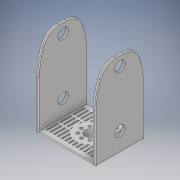
# Autodesk Inventor part: Wheel Case V3
Saved by Autodesk Inventor 2019 (Build 230136000, 136)
## iProperties
Created: 2018-12-01
Part Number: Wheel Case V3
Material: Generic
Document SubType Name: Modeling
Designer: Ashley
Density: 1 g/cm^3
Appearance: Default
Author: Ashley
Autodesk Inventor part; units mm, degrees
ref_plane "YZ Plane" through (0, 0, 0) normal (1, 0, 0) x (0, 1, 0)
ref_plane "XZ Plane" through (0, 0, 0) normal (0, 1, 0) x (-1, 0, 0)
ref_plane "XY Plane" through (0, 0, 0) normal (0, 0, 1) x (1, 0, 0)
sketch "Sketch1" plane through (0, 0, 0) normal (0, 1, 0) x (-1, 0, 0)
  line L0 (40, 32.5) -> (-40, 32.5)
  line L1 (-40, 32.5) -> (-40, -32.5)
  line L2 (-40, -32.5) -> (40, -32.5)
  line L3 (40, -32.5) -> (40, 32.5)
  line L4 (40, 32.5) -> (-40, -32.5) construction
  line L5 (-40, 32.5) -> (40, -32.5) construction
  point P0 (0, 0)
  dimension "d0" = 80
  dimension "d1" = 65
  constraints: 12 end point, 2 midpoint, 2 parallel, 1 horizontal, 1 perpendicular
  measures "d0" distance of L1.end L2.end
  measures "d1" distance of L0.end L1.end
extrude "Top Base Extrusion" add sketch "Sketch1" along normal blind 4
sketch "Sketch2" plane through (0, 4, 0) normal (0, 1, 0) x (1, 0, 0)
  line L0 (-40, -32.5) -> (40, -32.5) construction
  line L1 (40, -32.5) -> (40, 32.5) construction
  line L2 (-40, 32.5) -> (-40, -32.5) construction
  line L3 (-40, 32.5) -> (-36, 32.5)
  line L4 (-36, 32.5) -> (-36, -32.5)
  line L5 (-36, -32.5) -> (-40, -32.5)
  line L6 (-40, -32.5) -> (-40, 32.5)
  line L7 (40, 32.5) -> (36, 32.5)
  line L8 (36, 32.5) -> (36, -32.5)
  line L9 (36, -32.5) -> (40, -32.5)
  line L10 (40, -32.5) -> (40, 32.5)
  point P0 (0, 0)
  dimension "d4" = 4
  dimension "d5" = 4
  constraints: 16 end point, 4 parallel, 2 horizontal, 2 perpendicular, 2 point on line
  measures "d4" distance between parallel lines of L4 L2
  measures "d5" distance between parallel lines of L1 L8
extrude "Side Extrusions" add sketch "Sketch2" along normal blind 110
sketch "Sketch3" plane through (40, 0, 32.5) normal (1, 0, 0) x (0, 0, -1)
  circle A0 centre (32.5, 101.5) radius 7.1
  circle A1 centre (32.5, 26.5) radius 7
  line L0 (65, 0) -> (65, 114) construction
  line L1 (0, 114) -> (65, 114) construction
  line L2 (0, 0) -> (0, 114) construction
  line L3 (0, 4) -> (65, 4) construction
  point P0 (32.5, 0)
  dimension "d8" = 14.2
  dimension "d11" = 101.5
  dimension "d43" = 75
  dimension "d44" = 14
  dimension "d45" = 65
  dimension "d46" = 32.5
  dimension "d47" = 32.5
  dimension "d48" = 32.5
  dimension "d49" = 12.5
  dimension "d50" = 22.5
  constraints: 2 centre point
  measures "d8" diameter of A0
  measures "d11" distance of point (32.5, 0) A0.centre
  measures "d43" distance of A1.centre A0.centre
  measures "d44" diameter of A1
  measures "d45" distance between parallel lines of L2 L0
  measures "d46" distance from line of L0 A0.centre
  measures "d47" distance from line of L2 A0.centre
  measures "d48" distance from line of L0 A1.centre
  measures "d49" distance from line of A0.centre L1
  measures "d50" distance from line of A1.centre L3
extrude "Wheel Axel Hole" cut sketch "Sketch3" against normal up to surface (80 mm away)
sketch "Sketch4" plane through (0, 0, 0) normal (0, -1, 0) x (1, 0, 0)
  circle A0 centre (0, 0) radius 7.1
  circle A1 centre (0, 0) radius 16
  dimension "d16" = 14.2
  dimension "d17" = 32
  constraints: 2 centre point, 2 coincident
  measures "d16" diameter of A0
  measures "d17" diameter of A1
extrude "Chain Interferance Extrusion" add sketch "Sketch4" along normal blind 6
sketch "Sketch5" plane through (0, 0, 0) normal (0, -1, 0) x (1, 0, 0)
  circle A0 centre (0, 0) radius 7.1 construction
  circle A1 centre (0, 0) radius 7.1
  constraints: 1 centre point, 1 coincident, 1 concentric
extrude "Top Center Bearing Hole" cut sketch "Sketch5" against normal up to surface (4 mm away)
sketch "Sketch7" plane through (0, -6, 0) normal (0, -1, 0) x (1, 0, 0)
  circle A0 centre (0, 0) radius 7.1 construction
  circle A1 centre (0, 11.314) radius 2.05
  circle A2 centre (-8.0002, 8.0002) radius 2.05
  circle A3 centre (-11.314, 0) radius 2.05
  circle A4 centre (-8.0002, -8.0002) radius 2.05
  circle A5 centre (0, -11.314) radius 2.05
  circle A6 centre (8.0002, -8.0002) radius 2.05
  circle A7 centre (11.314, 0) radius 2.05
  circle A8 centre (8.0002, 8.0002) radius 2.05
  dimension "d23" = 4.1
  dimension "d24" = 11.314
  dimension "d27" = 360
  constraints: 8 centre point, 17 other
  measures "d23" diameter of A1
  measures "d24" distance of A0.centre A1.centre
extrude "Sprocket Screws Holes" cut sketch "Sketch7" against normal up to next
sketch "Sketch8" plane through (40, 0, 32.5) normal (1, 0, 0) x (0, 0, -1)
  line L0 (65, 0) -> (65, 114) construction
  line L1 (0, 114) -> (65, 114) construction
  line L2 (0, 0) -> (0, 114) construction
  line L3 (65, 91.5) -> (52.0096, 114)
  line L4 (65, 114) -> (0, 114) construction
  line L5 (65, 91.5) -> (90.9808, 91.5) construction
  line L6 (0, 91.5) -> (34.6363, 91.5) construction
  line L7 (0, 91.5) -> (44.4453, 91.5) construction
  line L8 (0, 91.5) -> (12.9904, 114)
  line L9 (65, 91.5) -> (65, 114)
  line L10 (52.0096, 114) -> (65, 114)
  line L11 (12.9904, 114) -> (0, 114)
  line L12 (0, 91.5) -> (0, 114)
  line L13 (0, 91.5) -> (-31.251, 91.5) construction
  point P0 (32.5, 0)
  dimension "d32" = 120
  dimension "d51" = 120
  constraints: 20 end point, 5 point on line, 3 collinear, 3 horizontal, 1 equal length, 1 perpendicular
  measures "d32" angle of L5 L3
  measures "d51" angle of L13 L8
extrude "Side Corners Cut" cut sketch "Sketch8" against normal up to surface (80 mm away)
fillet "Fillet1" radius 95 4 edges at (38, 91.5, 32.5) (-38, 91.5, 32.5) (38, 91.5, -32.5) (-38, 91.5, -32.5)
fillet "Fillet2" radius 23 4 edges at (38, 114, 19.5096) (38, 114, -19.5096) (-38, 114, -19.5096) (-38, 114, 19.5096)
fillet "Fillet3" radius 3 4 edges at (0, 0, -32.5) (-40, 0, 0) (40, 0, 0) (0, 0, 32.5)
fillet "Fillet4" radius 3 1 edges at (-16, 0, 0)
fillet "Fillet5" radius 1 1 edges at (-16, -6, 0)
fillet "Fillet7" radius 1 34 edges at (40, 109.8726, 18.1832) (40, 114, 0) (40, 109.8726, -18.1832) (40, 82.7695, -31.0162) (40, 34.5224, -32.5) (39.1213, 0.8787, -31.6213) (40, 34.5224, 32.5) (39.1213, 0.8787, 31.6213) (40, 82.7695, 31.0162) (36, 35.0224, 32.5) (36, 109.8726, 18.1832) (36, 114, 0) (36, 109.8726, -18.1832) (36, 82.7695, -31.0162) (36, 35.0224, -32.5) (36, 82.7695, 31.0162) (-36, 109.8726, 18.1832) (-36, 114, 0) (-36, 109.8726, -18.1832) (-36, 82.7695, -31.0162) (-36, 35.0224, -32.5) (-36, 35.0224, 32.5) (-36, 82.7695, 31.0162) (-40, 34.5224, 32.5) (-39.1213, 0.8787, 31.6213) (-40, 109.8726, 18.1832) (-40, 114, 0) (-40, 109.8726, -18.1832) (-40, 82.7695, -31.0162) (-40, 34.5224, -32.5) (-39.1213, 0.8787, -31.6213) (-40, 82.7695, 31.0162) (0, 4, 32.5) (0, 4, -32.5)
sketch "Sketch10" plane through (0, 0, 0) normal (0, -1, 0) x (1, 0, 0)
  line L0 (-37, 29.5) -> (37, 29.5) construction
  line L1 (-37, -29.5) -> (-37, 29.5) construction
  line L2 (37, -29.5) -> (-37, -29.5) construction
  line L3 (37, 29.5) -> (37, -29.5) construction
  circle A0 centre (0, 0) radius 19 construction
  line L4 (33.5, -25.5) -> (31.5, -25.5)
  line L5 (31.5, -25.5) -> (31.5, -10.5)
  line L6 (31.5, -10.5) -> (33.5, -10.5)
  line L7 (33.5, -10.5) -> (33.5, -25.5)
  line L8 (31.5, -7.5) -> (31.5, 7.5)
  line L9 (33.5, 7.5) -> (33.5, -7.5)
  line L10 (31.5, 7.5) -> (33.5, 7.5)
  line L11 (33.5, -7.5) -> (31.5, -7.5)
  line L12 (31.5, 10.5) -> (31.5, 25.5)
  line L13 (33.5, 25.5) -> (33.5, 10.5)
  line L14 (31.5, 25.5) -> (33.5, 25.5)
  line L15 (33.5, 10.5) -> (31.5, 10.5)
  line L16 (26.5, -25.5) -> (26.5, -10.5)
  line L17 (28.5, -10.5) -> (28.5, -25.5)
  line L18 (26.5, -10.5) -> (28.5, -10.5)
  line L19 (28.5, -25.5) -> (26.5, -25.5)
  line L20 (26.5, -7.5) -> (26.5, 7.5)
  line L21 (28.5, 7.5) -> (28.5, -7.5)
  line L22 (26.5, 7.5) -> (28.5, 7.5)
  line L23 (28.5, -7.5) -> (26.5, -7.5)
  line L24 (26.5, 10.5) -> (26.5, 25.5)
  line L25 (28.5, 25.5) -> (28.5, 10.5)
  line L26 (26.5, 25.5) -> (28.5, 25.5)
  line L27 (28.5, 10.5) -> (26.5, 10.5)
  line L28 (21.5, -25.5) -> (21.5, -10.5)
  line L29 (23.5, -10.5) -> (23.5, -25.5)
  line L30 (21.5, -10.5) -> (23.5, -10.5)
  line L31 (23.5, -25.5) -> (21.5, -25.5)
  line L32 (21.5, -7.5) -> (21.5, 7.5)
  line L33 (23.5, 7.5) -> (23.5, -7.5)
  line L34 (21.5, 7.5) -> (23.5, 7.5)
  line L35 (23.5, -7.5) -> (21.5, -7.5)
  line L36 (21.5, 10.5) -> (21.5, 25.5)
  line L37 (23.5, 25.5) -> (23.5, 10.5)
  line L38 (21.5, 25.5) -> (23.5, 25.5)
  line L39 (23.5, 10.5) -> (21.5, 10.5)
  line L40 (16.5, -25.5) -> (16.5, -10.5)
  line L41 (18.5, -10.5) -> (18.5, -25.5)
  line L42 (16.5, -10.5) -> (18.5, -10.5)
  line L43 (18.5, -25.5) -> (16.5, -25.5)
  line L44 (16.5, 10.5) -> (16.5, 25.5)
  line L45 (16.5, 25.5) -> (18.5, 25.5)
  line L46 (18.5, 10.5) -> (16.5, 10.5)
  line L47 (18.5, 25.5) -> (18.5, 10.5)
  line L48 (13.5, 25.5) -> (11.5, 25.5)
  line L49 (11.5, 25.5) -> (11.5, 15.1245)
  line L50 (13.5, 13.3697) -> (13.5, 25.5)
  line L51 (8.5, 25.5) -> (6.5, 25.5)
  line L52 (6.5, 25.5) -> (6.5, 17.8536)
  line L53 (8.5, 16.9926) -> (8.5, 25.5)
  line L54 (3.5, 25.5) -> (1.5, 25.5)
  line L55 (1.5, 25.5) -> (1.5, 18.9407)
  line L56 (3.5, 18.6748) -> (3.5, 25.5)
  line L57 (-1.5, 25.5) -> (-3.5, 25.5)
  line L58 (-3.5, 25.5) -> (-3.5, 18.6748)
  line L59 (-1.5, 18.9407) -> (-1.5, 25.5)
  line L60 (-6.5, 25.5) -> (-8.5, 25.5)
  line L61 (-8.5, 25.5) -> (-8.5, 16.9926)
  line L62 (-6.5, 17.8536) -> (-6.5, 25.5)
  line L63 (-11.5, 25.5) -> (-13.5, 25.5)
  line L64 (-13.5, 25.5) -> (-13.5, 13.3697)
  line L65 (-11.5, 15.1245) -> (-11.5, 25.5)
  line L66 (-16.5, 25.5) -> (-18.5, 25.5)
  line L67 (-18.5, 25.5) -> (-18.5, 10.5)
  line L68 (-13, 10.5) -> (-11, 10.5)
  line L69 (-16.5, 10.5) -> (-16.5, 25.5)
  line L70 (41.0278, 0) -> (-51.455, 0) construction
  line L71 (-16.5, 10.5) -> (-18.5, 10.5)
  line L72 (-21.5, 25.5) -> (-23.5, 25.5)
  line L73 (-21.5, 10.5) -> (-21.5, 25.5)
  line L74 (-23.5, 25.5) -> (-23.5, 10.5)
  line L75 (-21.5, 10.5) -> (-23.5, 10.5)
  line L76 (-26.5, 25.5) -> (-28.5, 25.5)
  line L77 (-26.5, 10.5) -> (-26.5, 25.5)
  line L78 (-28.5, 25.5) -> (-28.5, 10.5)
  line L79 (-26.5, 10.5) -> (-28.5, 10.5)
  line L80 (-31.5, 25.5) -> (-33.5, 25.5)
  line L81 (-31.5, 10.5) -> (-31.5, 25.5)
  line L82 (-33.5, 25.5) -> (-33.5, 10.5)
  line L83 (-31.5, 10.5) -> (-33.5, 10.5)
  line L84 (-16.5, 0) -> (-16.5, -0.9905)
  line L85 (-18.5, 4.3301) -> (-18.5, 7.5)
  line L86 (-21.5, -7.5) -> (-21.5, 7.5)
  line L87 (-21.5, -7.5) -> (-23.5, -7.5)
  line L88 (-23.5, 7.5) -> (-23.5, -7.5)
  line L89 (-21.5, 7.5) -> (-23.5, 7.5)
  line L90 (-18.5, 7.5) -> (-17.4571, 7.5)
  line L91 (36.0278, 0) -> (-56.455, 0) construction
  line L92 (-28.5, 7.5) -> (-28.5, -7.5)
  line L93 (-26.5, -7.5) -> (-26.5, 7.5)
  line L94 (-26.5, 7.5) -> (-28.5, 7.5)
  line L95 (-26.5, -7.5) -> (-28.5, -7.5)
  line L96 (31.0278, 0) -> (-61.455, 0) construction
  line L97 (-33.5, 7.5) -> (-33.5, -7.5)
  line L98 (-31.5, -7.5) -> (-31.5, 7.5)
  line L99 (-31.5, 7.5) -> (-33.5, 7.5)
  line L100 (-31.5, -7.5) -> (-33.5, -7.5)
  line L101 (41.0278, -18) -> (-51.455, -18) construction
  line L102 (-23.5, -10.5) -> (-23.5, -25.5)
  line L103 (-21.5, -25.5) -> (-21.5, -10.5)
  line L104 (-21.5, -10.5) -> (-23.5, -10.5)
  line L105 (-21.5, -25.5) -> (-23.5, -25.5)
  line L106 (36.0278, -18) -> (-56.455, -18) construction
  line L107 (-28.5, -10.5) -> (-28.5, -25.5)
  line L108 (-26.5, -25.5) -> (-26.5, -10.5)
  line L109 (-26.5, -10.5) -> (-28.5, -10.5)
  line L110 (-26.5, -25.5) -> (-28.5, -25.5)
  line L111 (31.0278, -18) -> (-61.455, -18) construction
  line L112 (-33.5, -10.5) -> (-33.5, -25.5)
  line L113 (-31.5, -25.5) -> (-31.5, -10.5)
  line L114 (-31.5, -10.5) -> (-33.5, -10.5)
  line L115 (-31.5, -25.5) -> (-33.5, -25.5)
  line L116 (-16.5, -25.5) -> (-18.5, -25.5)
  line L117 (-16.5, -25.5) -> (-16.5, -10.5)
  line L118 (-18.5, -10.5) -> (-18.5, -25.5)
  line L119 (-16.5, -10.5) -> (-18.5, -10.5)
  arc A1 (-17.4571, 7.5) -> (-18.5, 4.3301) centre (0, 0) ccw
  line L120 (-18.5, -4.3301) -> (-18.5, -7.5)
  line L121 (-18.5, -7.5) -> (-17.4571, -7.5)
  arc A2 (-18.5, -4.3301) -> (-17.4571, -7.5) centre (0, 0) ccw
  arc A3 (-11.5, 15.1245) -> (-13.5, 13.3697) centre (0, 0) ccw
  arc A4 (-6.5, 17.8536) -> (-8.5, 16.9926) centre (0, 0) ccw
  arc A5 (-1.5, 18.9407) -> (-3.5, 18.6748) centre (0, 0) ccw
  arc A6 (3.5, 18.6748) -> (1.5, 18.9407) centre (0, 0) ccw
  arc A7 (8.5, 16.9926) -> (6.5, 17.8536) centre (0, 0) ccw
  line L122 (18.5, 7.5) -> (17.4571, 7.5)
  line L123 (18.5, 4.3301) -> (18.5, 7.5)
  arc A8 (18.5, 4.3301) -> (17.4571, 7.5) centre (0, 0) ccw
  arc A9 (13.5, 13.3697) -> (11.5, 15.1245) centre (0, 0) ccw
  line L124 (13.5, -25.5) -> (11.5, -25.5)
  line L125 (11.5, -25.5) -> (11.5, -15.1245)
  line L126 (13.5, -13.3697) -> (13.5, -25.5)
  line L127 (8.5, -25.5) -> (6.5, -25.5)
  line L128 (6.5, -25.5) -> (6.5, -17.8536)
  line L129 (8.5, -16.9926) -> (8.5, -25.5)
  line L130 (3.5, -25.5) -> (1.5, -25.5)
  line L131 (1.5, -25.5) -> (1.5, -18.9407)
  line L132 (3.5, -18.6748) -> (3.5, -25.5)
  line L133 (-1.5, -25.5) -> (-3.5, -25.5)
  line L134 (-3.5, -25.5) -> (-3.5, -18.6748)
  line L135 (-1.5, -18.9407) -> (-1.5, -25.5)
  line L136 (-6.5, -25.5) -> (-8.5, -25.5)
  line L137 (-8.5, -25.5) -> (-8.5, -16.9926)
  line L138 (-6.5, -17.8536) -> (-6.5, -25.5)
  line L139 (-11.5, -25.5) -> (-13.5, -25.5)
  line L140 (-13.5, -25.5) -> (-13.5, -13.3697)
  line L141 (-11.5, -15.1245) -> (-11.5, -25.5)
  arc A10 (-13.5, -13.3697) -> (-11.5, -15.1245) centre (0, 0) ccw
  arc A11 (-8.5, -16.9926) -> (-6.5, -17.8536) centre (0, 0) ccw
  arc A12 (-3.5, -18.6748) -> (-1.5, -18.9407) centre (0, 0) ccw
  arc A13 (1.5, -18.9407) -> (3.5, -18.6748) centre (0, 0) ccw
  arc A14 (6.5, -17.8536) -> (8.5, -16.9926) centre (0, 0) ccw
  line L142 (18.5, -7.5) -> (17.4571, -7.5)
  line L143 (18.5, -4.3301) -> (18.5, -7.5)
  arc A15 (17.4571, -7.5) -> (18.5, -4.3301) centre (0, 0) ccw
  arc A16 (11.5, -15.1245) -> (13.5, -13.3697) centre (0, 0) ccw
  point P0 (-19, 0)
  point P1 (19, 0)
  point P2 (-24, 0)
  point P3 (14, 0)
  point P4 (-21.5, 0)
  point P5 (-29, 0)
  point P6 (9, 0)
  point P7 (-26.5, 0)
  point P8 (-19, -18)
  point P9 (19, -18)
  point P10 (-16.5, -18)
  point P11 (-24, -18)
  point P12 (14, -18)
  point P13 (-21.5, -18)
  point P14 (-29, -18)
  point P15 (9, -18)
  point P16 (-26.5, -18)
  dimension "d175" = 2
  dimension "d176" = 15
  dimension "d177" = 4
  dimension "d178" = 3.5
  dimension "d181" = 18
  dimension "d184" = 5
  dimension "d187" = 4
  dimension "d190" = 5
  dimension "d197" = 5
  dimension "d203" = 3
  dimension "d204" = 2
  dimension "d205" = 2
  dimension "d206" = 3
  dimension "d207" = 2
  dimension "d208" = 3
  dimension "d209" = 2
  dimension "d210" = 3
  dimension "d211" = 3
  dimension "d212" = 2
  dimension "d213" = 3
  dimension "d214" = 2
  dimension "d216" = 2
  dimension "d217" = 3
  dimension "d219" = 15
  dimension "d222" = 5
  dimension "d227" = 3.5
  dimension "d230" = 18
  dimension "d235" = 3
  dimension "d237" = 3
  dimension "d239" = 3
  dimension "d242" = 5
  dimension "d245" = 18
  dimension "d250" = 5
  dimension "d255" = 3
  dimension "d256" = 3
  constraints: 280 end point, 32 point on circle, 30 symmetric about line, 18 point on line, 17 horizontal, 16 centre point, 11 parallel, 9 perpendicular, 3 vertical, 1 coincident, 198 other
  measures "d175" distance of L5.end L6.end
  measures "d176" distance of L4.end L5.end
  measures "d177" distance between parallel lines of L4 L2
  measures "d178" distance between parallel lines of L3 L7
  measures "d181" distance of L4.end L8.start
  measures "d184" distance of L4.end L16.start
  measures "d187" distance between parallel lines of L0 L14
  measures "d190" distance of L28.start L40.start
  measures "d197" distance of L36.start L44.start
  measures "d203" distance between parallel lines of L50 L44
  measures "d204" distance of L48.start L48.end
  measures "d205" distance of L51.start L51.end
  measures "d206" distance between parallel lines of L53 L49
  measures "d207" distance of L54.start L54.end
  measures "d208" distance between parallel lines of L56 L52
  measures "d209" distance of L57.start L57.end
  measures "d210" distance between parallel lines of L55 L59
  measures "d211" distance between parallel lines of L58 L62
  measures "d212" distance of L60.start L60.end
  measures "d213" distance between parallel lines of L61 L65
  measures "d214" distance between parallel lines of L64 L65
  measures "d216" distance of L66.start L66.end
  measures "d217" distance between parallel lines of L64 L69
  measures "d219" distance between parallel lines of L66 L71
  measures "d222" distance of L66.start L72.start
  measures "d227" distance between parallel lines of L1 L82
  measures "d230" distance of L72.start L86.end
  measures "d235" distance between parallel lines of L39 L34
  measures "d237" distance between parallel lines of L71 L90
  measures "d239" distance between parallel lines of L86 L85
  measures "d242" distance of L70.start L91.start
  measures "d245" distance of L70.start L101.start
  measures "d250" distance of L103.start L116.start
  measures "d255" distance between parallel lines of L32 L123
  measures "d256" distance between parallel lines of L46 L122
extrude "Extrusion9" cut sketch "Sketch10" against normal up to surface (4 mm away)
body "Solid1"
